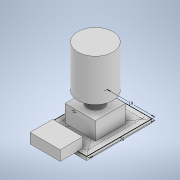
# Autodesk Inventor part: encoder_footprint
Saved by Autodesk Inventor 2021 (Build 250183000, 183)
## iProperties
Created: 2021-12-12
Part Number: encoder_footprint
Material: Generic
Document SubType Name: Modeling
Designer: Juan M. Casillas
Density: 1 g/cm^3
Appearance: Default
Author: Juan M. Casillas
Autodesk Inventor part; units mm, degrees
ref_plane "YZ Plane" through (0, 0, 0) normal (1, 0, 0) x (0, 1, 0)
ref_plane "XZ Plane" through (0, 0, 0) normal (0, 1, 0) x (-1, 0, 0)
ref_plane "XY Plane" through (0, 0, 0) normal (0, 0, 1) x (1, 0, 0)
sketch "Sketch1" plane through (0, 0, 0) normal (0, 1, 0) x (-1, 0, 0)
  line L0 (9.5, 13) -> (-9.5, 13)
  line L1 (-9.5, 13) -> (-9.5, -13)
  line L2 (-9.5, -13) -> (9.5, -13)
  line L3 (9.5, -13) -> (9.5, 13)
  line L4 (9.5, 13) -> (-9.5, -13) construction
  line L5 (-9.5, 13) -> (9.5, -13) construction
  line L6 (7.5, 11) -> (-7.5, 11) construction
  line L7 (-7.5, 11) -> (-7.5, -11) construction
  line L8 (-7.5, -11) -> (7.5, -11) construction
  line L9 (7.5, -11) -> (7.5, 11) construction
  point P0 (0, 0)
  dimension "d0" = 19
  dimension "d1" = 26
  dimension "d2" = 2
  constraints: 20 end point, 4 parallel, 3 coincident, 2 midpoint, 2 perpendicular, 1 horizontal, 3 other
  measures "d0" distance of L2.end L1.end
  measures "d1" distance of L1.end L0.end
  measures "d2" distance between parallel lines of L3 L9
extrude "Extrusion1" add sketch "Sketch1" against normal blind 1.5
sketch "Sketch2" plane through (0, 0, 0) normal (0, 1, 0) x (1, 0, 0)
  line L0 (-6, -19.9878) -> (6, -19.9878)
  line L1 (6, -19.9878) -> (6, -10.9878)
  line L2 (6, -10.9878) -> (-6, -10.9878)
  line L3 (-6, -10.9878) -> (-6, -19.9878)
  line L4 (-6, -19.9878) -> (6, -10.9878) construction
  line L5 (6, -19.9878) -> (-6, -10.9878) construction
  line L6 (-9.5, 13) -> (-9.5, -13) projected
  line L7 (-9.5, -13) -> (9.5, -13) projected
  point P0 (0, 0)
  point P1 (0, -15.4878)
  point P2 (0, -10.9878)
  point P3 (0, -10.9878)
  point P4 (0, -10.9878)
  dimension "d12" = 12
  dimension "d13" = 9
  dimension "d14" = 9.5
  dimension "d15" = 2.0122
  constraints: 12 end point, 3 midpoint, 2 coincident, 2 parallel, 1 horizontal, 1 perpendicular
  measures "d12" distance of L2.end L1.end
  measures "d13" distance of L1.end L0.end
  measures "d14" distance from line of L6 point (0, -10.988)
  measures "d15" distance from line of L7 point (0, -10.988)
extrude "Extrusion2" add sketch "Sketch2" along normal blind 4
sketch "Sketch3" plane through (0, 0, 0) normal (0, 1, 0) x (1, 0, 0)
  line L0 (-6, -6) -> (6, -6)
  line L1 (6, -6) -> (6, 6)
  line L2 (6, 6) -> (-6, 6)
  line L3 (-6, 6) -> (-6, -6)
  line L4 (-6, -6) -> (6, 6) construction
  line L5 (6, -6) -> (-6, 6) construction
  point P0 (0, 0)
  dimension "d18" = 12
  dimension "d19" = 12
  constraints: 12 end point, 2 midpoint, 2 parallel, 1 horizontal, 1 perpendicular
  measures "d18" distance of L2.end L1.end
  measures "d19" distance of L1.end L0.end
hole "Hole2" at (-7.5, 0, 11) at (-7.5, 0, -11) direction (0, -1, 0) diameter 3 end through all
extrude "Extrusion3" add sketch "Sketch3" along normal blind 7
sketch "Sketch4" plane through (0, 7, 0) normal (0, 1, 0) x (1, 0, 0)
  circle A0 centre (0, 0) radius 3.25
  dimension "d29" = 6.5
  constraints: 1 centre point, 1 coincident
  measures "d29" diameter of A0
extrude "Extrusion4" add sketch "Sketch4" along normal blind 4.5
sketch "Sketch5" plane through (0, 11.5, 0) normal (0, 1, 0) x (1, 0, 0)
  circle A0 centre (0, 0) radius 7
  dimension "d32" = 14
  constraints: 1 centre point, 1 coincident
  measures "d32" diameter of A0
extrude "Extrusion5" add sketch "Sketch5" along normal blind 16.7
body "Solid1"
